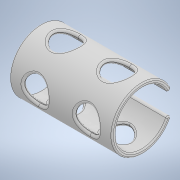
# Autodesk Inventor part: Cable_Ring
Saved by Autodesk Inventor 2020 (Build 240168000, 168)
## iProperties
Created: 2020-09-22
Part Number: Cable_Ring
Material: Generic
Document SubType Name: Modeling
Designer: maple
Density: 1 g/cm^3
Appearance: Default
Author: maple
Autodesk Inventor part; units mm, degrees
ref_plane "YZ Plane" through (0, 0, 0) normal (1, 0, 0) x (0, 1, 0)
ref_plane "XZ Plane" through (0, 0, 0) normal (0, 1, 0) x (-1, 0, 0)
ref_plane "XY Plane" through (0, 0, 0) normal (0, 0, 1) x (1, 0, 0)
sketch "Sketch1" plane through (0, 0, 0) normal (1, 0, 0) x (0, 1, 0)
  circle A0 centre (0, 0) radius 15
  line L0 (15, 0) -> (13, 0)
  circle A1 centre (0, 0) radius 13
  line L1 (0, -13) -> (0, -15)
  circle A2 centre (0, 0) radius 14
  line L2 (0, 0) -> (5.1303, -14.0954)
  line L3 (0, 0) -> (15, 0) construction
  line L4 (0, 0) -> (-5.1303, -14.0954)
  line L5 (4.4463, -12.216) -> (4.2753, -11.7462)
  line L6 (5.1303, -14.0954) -> (5.3013, -14.5652)
  line L7 (-4.4463, -12.216) -> (-4.2753, -11.7462)
  line L8 (-5.1303, -14.0954) -> (-5.3013, -14.5652)
  circle A3 centre (0, 0) radius 12.5
  circle A4 centre (0, 0) radius 15.5
  line L9 (4.2753, -11.7462) -> (3.7622, -10.3366)
  line L10 (5.3013, -14.5652) -> (5.8143, -15.9748)
  line L11 (-4.2753, -11.7462) -> (-3.7622, -10.3366)
  line L12 (-5.3013, -14.5652) -> (-5.8143, -15.9748)
  circle A5 centre (0, 0) radius 11
  circle A6 centre (0, 0) radius 17
  line L13 (3.7622, -10.3366) -> (7.0288, -10.3366)
  line L14 (7.0288, -10.3366) -> (6.1854, -9.0962)
  line L15 (-3.7622, -10.3366) -> (-7.0288, -10.3366)
  line L16 (-7.0288, -10.3366) -> (-6.1854, -9.0962)
  line L17 (6.1854, -9.0962) -> (9.5592, -14.0578)
  line L18 (-6.1854, -9.0962) -> (-9.5592, -14.0578)
  line L19 (4.4463, -12.216) -> (4.9127, -12.036)
  line L20 (5.1303, -14.0954) -> (5.5972, -13.9166)
  line L21 (5.5972, -13.9166) -> (4.9127, -12.036)
  line L22 (-5.1303, -14.0954) -> (-5.5972, -13.9166)
  line L23 (-4.4463, -12.216) -> (-4.9127, -12.036)
  line L24 (-4.9127, -12.036) -> (-5.5972, -13.9166)
  dimension "d0" = 30
  dimension "d1" = 2
  dimension "d2" = 70
  dimension "d3" = 0.5
  dimension "d4" = 0.5
  dimension "d5" = 0.5
  dimension "d6" = 0.5
  dimension "d7" = 1.5
  dimension "d8" = 1.5
  dimension "d9" = 1.5
  dimension "d10" = 1.5
  dimension "d11" = 1.5
  dimension "d12" = 1.5
  dimension "d13" = 0.5
  dimension "d14" = 0.5
  dimension "d15" = 0.5
  dimension "d16" = 0.5
  constraints: 50 end point, 15 point on circle, 7 coincident, 7 point on line, 5 centre point, 4 horizontal, 1 equal length, 1 vertical, 12 other
  measures "d0" diameter of A0
  measures "d1" distance of L0.start L0.end
  measures "d2" angle of L2 L3
  measures "d3" distance of L5.start L5.end
  measures "d4" distance of L2.end L6.end
  measures "d5" distance of L7.start L7.end
  measures "d6" distance of L4.end L8.end
  measures "d7" distance of L5.end L9.end
  measures "d8" distance of L6.end L10.end
  measures "d9" distance of L7.end L11.end
  measures "d10" distance of L8.end L12.end
  measures "d11" distance of L13.end L14.end
  measures "d12" distance of L15.end L16.end
  measures "d13" distance of L19.start L19.end
  measures "d14" distance of L2.end L20.end
  measures "d15" distance of L4.end L22.end
  measures "d16" distance of L7.start L23.end
extrude "Extrusion1" add sketch "Sketch1" along normal blind 50 contours A0 L18 A2 L24 | A0 L0 A2 L18 | A2 L18 A1 L24 | A0 L17 A2 L0 | A2 L0 A1 L18 | A0 L21 A2 L17 | A2 L17 A1 L0 | A2 L21 A1 L17
sketch "Sketch2" plane through (0, 0, 0) normal (0, 1, 0) x (-1, 0, 0)
  line L0 (-50, 15) -> (-50, -13.9166) projected
  line L1 (-50, 0) -> (0, 0)
  line L2 (-25, 0) -> (0, 0)
  line L3 (0, 15) -> (0, -13.9166) projected
  line L4 (-25, 0) -> (-50, 0)
  circle A0 centre (-12.5, 0) radius 6
  circle A1 centre (-37.5, 0) radius 6
  dimension "d19" = 12
  dimension "d20" = 12
  constraints: 6 end point, 3 midpoint, 2 centre point, 1 collinear, 1 horizontal, 1 perpendicular, 1 point on line
  measures "d19" diameter of A0
  measures "d20" diameter of A1
extrude "Extrusion2" cut sketch "Sketch2" against normal mid plane 50
sketch "Sketch3" plane through (0, 0, 0) normal (0, 0, 1) x (1, 0, 0)
  line L0 (0, 0) -> (50, 0)
  line L1 (50, 13) -> (50, -13) projected
  line L2 (50, 0) -> (25, 0)
  line L3 (0, 0) -> (25, 0)
  circle A0 centre (37.5, 0) radius 6
  circle A1 centre (12.5, 0) radius 6
  point P0 (50, -4.9127)
  point P1 (50, 4.9127)
  dimension "d23" = 12
  dimension "d24" = 12
  constraints: 6 end point, 4 midpoint, 2 centre point, 1 collinear
  measures "d23" diameter of A0
  measures "d24" diameter of A1
extrude "Extrusion3" cut sketch "Sketch3" along normal blind 50
fillet "Fillet1" radius 1 4 edges at (25, 5.5972, -13.9166) (25, 4.9127, -12.036) (25, -4.9127, -12.036) (25, -5.5972, -13.9166)
fillet "Fillet2" radius 0.9 12 edges at (43.5, -13, -0.0106) (43.5, 13, -0.0106) (43.5, -15, 0.0093) (43.5, 15, 0.0093) (18.5, -15, 0.0093) (18.5, 15, 0.0093) (18.5, -13, -0.0106) (18.5, 13, -0.0106) (6.5, -0.0079, 13) (6.5, -0.0013, 15) (31.5, -0.0079, 13) (31.5, -0.0013, 15)
fillet "Fillet3" radius 0.6 8 edges at (50, -5.2424, -12.1935) (50, 0, 13) (50, 5.7967, -13.4949) (50, 0, 15) (0, 5.7967, -13.4949) (0, 0, 15) (0, -5.2424, -12.1935) (0, 0, 13)
body "Solid1"
